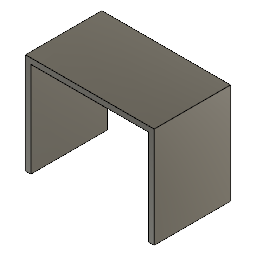
CAD FILE_ (Autodesk Fusion 360 archive; units mm, degrees)
design "u"
Autodesk Fusion 360 part; units mm, degrees
box "BoxPrimitive1" add length 5 width 115 height 5 placed x (0, 0, -1) y (-1, 0, 0) z (0, 1, 0) at (80, 0, 15)
box "BoxPrimitive2" add length 85 width 5 height 5 placed x (0, 0, -1) y (-1, 0, 0) z (0, 1, 0) at (-30, 0, 10)
sketch "Sketch3" plane through (0, 0, 0) normal (0, 1, 0) x (1, 0, 0)
box "BoxPrimitive3" add length 85 width 5 height 5 placed x (0, 0, -1) y (-1, 0, 0) z (0, 1, 0) at (80, 0, 10)
scale "Scale1" factor 0.8 about (75, 0, 10) bodies 1
extrude "Extrude1" add 1 faces at (47, 0, 12.6667) along direction (0, -1, 0) blind 25
extrude "Extrude2" add 1 faces at (47, -25, 12.6667) along direction (0, -1, 0) blind 10
scale "Scale2" factor 0.8 about (-9, -35, 10) bodies 1
scale "Scale3" factor 1.2 about (58.2, -35, 10) bodies 1
extrude "Extrude3" add 1 faces at (4.44, -35, 12.56) along direction (0, -1, 0) blind 15
